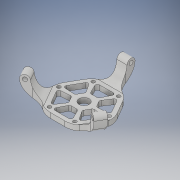
# Autodesk Inventor part: End_EffectorV2
Saved by Autodesk Inventor 2019.4 (Build 234330000, 330)
## iProperties
Created: 2020-01-10
Part Number: End_EffectorV2
Material: Generic
Document SubType Name: Modeling
Designer: Jorian Bruslind
Density: 1 g/cm^3
Appearance: Default
Author: Jorian Bruslind
Autodesk Inventor part; units mm, degrees
ref_plane "YZ Plane" through (0, 0, 0) normal (1, 0, 0) x (0, 1, 0)
ref_plane "XZ Plane" through (0, 0, 0) normal (0, 1, 0) x (-1, 0, 0)
sketch "Sketch1" plane through (0, 0, 0) normal (0, 1, 0) x (-1, 0, 0)
  line L0 (30, 0) -> (15, -25.9808)
  line L1 (15, -25.9808) -> (-15, -25.9808)
  line L2 (-15, -25.9808) -> (-30, 0)
  line L3 (-30, 0) -> (-15, 25.9808)
  line L4 (-15, 25.9808) -> (15, 25.9808)
  line L5 (15, 25.9808) -> (30, 0)
  point P0 (0, 0)
  point P1 (0, 0)
  dimension "d0" = 30
  dimension "d1" = 25.9808
  constraints: 12 end point, 1 coincident, 13 other
  measures "d0" distance of L0.end L1.end
  measures "d1" vertical distance of L4.end L0.start
extrude "Extrusion1" add sketch "Sketch1" along normal blind 5
ref_plane "Work Plane2" through (-22.5, 0, 12.9904) normal (0.5, 0, 0.8660254) x (0, 1, 0)
ref_plane "Work Plane1" through (-30, 0, 0) normal (0.5, 0, 0.8660254) x (0, 1, 0)
sketch "Sketch4" plane through (-22.5, 0, 12.9904) normal (0.5, 0, 0.8660254) x (0, 1, 0)
  line L0 (0, 0) -> (0, -25.9808) projected
  line L1 (0, 0) -> (0, 15.5)
  line L2 (0, 0) -> (15.5, 0) construction
  line L3 (0, 15.5) -> (20, 15.5)
  circle A0 centre (20, 15.5) radius 2
  circle A1 centre (20, 15.5) radius 4
  spline S0 degree 2 poles (0, 0) (7.2772, 18.8046) (20, 19.5) knots 0 0 0 1 1 1
  line L4 (5, -25.9808) -> (5, 0) projected
  spline S1 degree 2 poles (5, 0) (8.0439, 10.1774) (20, 11.5) knots 0 0 0 1 1 1
  line L5 (0, 0) -> (5, 0) projected
  line L6 (5, 0) -> (0, 0)
  point P0 (10, 15.5)
  point P1 (10.0001, 7.75)
  dimension "d15" = 15.5
  dimension "d16" = 90
  dimension "d17" = 20
  dimension "d18" = 90
  dimension "d19" = 4
  dimension "d20" = 8
  constraints: 8 end point, 2 centre point, 2 coincident, 2 perpendicular, 2 point on circle, 1 collinear, 1 horizontal, 1 midpoint, 1 vertical, 6 other
  measures "d15" distance of L0.start L1.end
  measures "d16" angle of L2 L1
  measures "d17" distance of L1.end L3.end
  measures "d18" angle of L1 L3
  measures "d19" diameter of A0
  measures "d20" diameter of A1
extrude "Extrusion3" add sketch "Sketch4" along normal mid plane 10 contours S0 L3 A1 S1 L5 | S0 A1 L3 | A1 S0 picked at (16.7043, 15.8146)
fillet "Fillet1" radius 10 2 edges at (-25, 2.5, 8.6603) (-20, 2.5, 17.3205)
sketch "Sketch5" plane through (0, 5, 0) normal (0, 1, 0) x (1, 0, 0)
  circle A0 centre (0, 0) radius 5
  dimension "d24" = 10
  constraints: 1 centre point, 1 coincident
  measures "d24" diameter of A0
extrude "Extrusion4" cut sketch "Sketch5" against normal blind 10
pattern_circular "Circular Pattern1" count 3 over 360 about axis through (0, 5, 0) along (0, -1, 0) of "Extrusion3"
fillet "Fillet2" radius 10 4 edges at (20, 2.5, 17.3205) (25, 2.5, 8.6603) (5, 2.5, -25.9808) (-5, 2.5, -25.9808)
sketch "Sketch6" plane through (0, 5, 0) normal (0, 1, 0) x (1, 0, 0)
  line L0 (-30, 0) -> (-15, 25.9808) projected
  line L1 (-30, 0) -> (-15, 25.9808)
  line L2 (-22.5, 12.9904) -> (-19.0359, 10.9904)
  line L3 (-22.5, 12.9904) -> (-18.5, 12.9904) construction
  line L4 (0, 0) -> (-15, 25.9808)
  line L5 (-19.0359, 10.9904) -> (-14.0359, 19.6506)
  line L6 (-19.0359, 10.9904) -> (-9.0359, 10.9904) construction
  line L7 (-19.0359, 10.9904) -> (-24.0359, 2.3301)
  line L8 (-19.0359, 10.9904) -> (-9.0359, 10.9904) construction
  line L9 (-19.0359, 10.9904) -> (-8.6436, 4.9904)
  line L10 (-19.0359, 10.9904) -> (-7.0359, 10.9904) construction
  line L11 (-8.6436, 4.9904) -> (-6.6436, 8.4545)
  line L12 (-8.6436, 4.9904) -> (-10.6436, 1.5263)
  line L13 (-10.6436, 1.5263) -> (-24.0359, 2.3301)
  line L14 (-6.6436, 8.4545) -> (-14.0359, 19.6506)
  dimension "d31" = 4
  dimension "d32" = 30
  dimension "d33" = 10
  dimension "d34" = 60
  dimension "d35" = 10
  dimension "d36" = 120
  dimension "d37" = 12
  dimension "d38" = 30
  dimension "d39" = 4
  dimension "d40" = 4
  constraints: 28 end point, 4 equal length, 4 horizontal, 2 perpendicular, 1 collinear, 1 midpoint, 1 parallel
  measures "d31" distance of L2.start L2.end
  measures "d32" angle of L2 L3
  measures "d33" distance of L2.end L5.end
  measures "d34" angle of L6 L5
  measures "d35" distance of L2.end L7.end
  measures "d36" angle of L7 L8
  measures "d37" distance of L2.end L9.end
  measures "d38" angle of L9 L10
  measures "d39" distance of L9.end L11.end
  measures "d40" distance of L9.end L12.end
extrude "Extrusion5" cut sketch "Sketch6" against normal blind 10
pattern_circular "Circular Pattern2" count 6 over 360 about axis through (0, 5, 0) along (0, -1, 0) of "Extrusion5"
fillet "Fillet3" radius 2 4 edges at (10, 2.5, -21.9808) (-10, 2.5, -21.9808) (4, 2.5, -9.9808) (-4, 2.5, -9.9808)
pattern_circular "Circular Pattern3" count 6 over 360 about axis through (0, 5, 0) along (0, -1, 0) of "Fillet3"
fillet "Fillet4" radius 20 6 edges at (30, 2.5, 0) (15, 2.5, 25.9808) (-15, 2.5, 25.9808) (15, 2.5, -25.9808) (-30, 2.5, 0) (-15, 2.5, -25.9808)
sketch "Sketch7" plane through (0, 5, 0) normal (0, 1, 0) x (1, 0, 0)
  line L0 (0, 0) -> (25, 0)
  circle A0 centre (25, 0) radius 1.75
  circle A1 centre (0, 0) radius 5
  circle A2 centre (12.5, 21.6506) radius 1.75
  circle A3 centre (-12.5, 21.6506) radius 1.75
  circle A4 centre (-25, 0) radius 1.75
  circle A5 centre (-12.5, -21.6506) radius 1.75
  circle A6 centre (12.5, -21.6506) radius 1.75
  dimension "d51" = 25
  dimension "d52" = 3.5
  dimension "d55" = 360
  constraints: 7 centre point, 2 coincident, 2 end point, 1 horizontal, 13 other
  measures "d51" distance of L0.start L0.end
  measures "d52" diameter of A0
extrude "Extrusion6" cut sketch "Sketch7" against normal blind 10 contours A0 | A2 | A3 | A4 | A5 | A6
body "Solid1"
